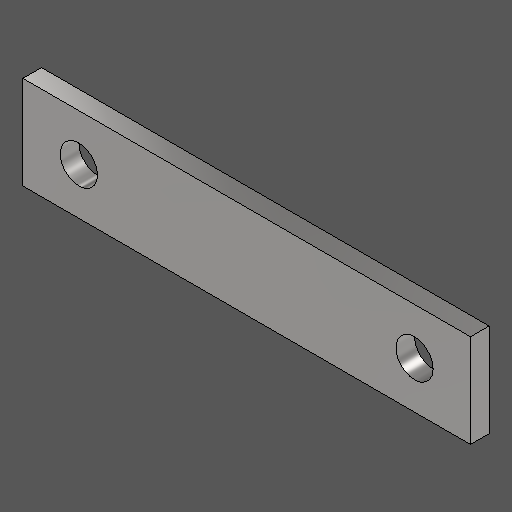
# Autodesk Inventor part: probe-side-large-mesh-support-plate
Saved by Autodesk Inventor 2025 (Build 290162000, 162)
## iProperties
Created: 2024-05-22
Part Number: probe-side-large-mesh-support-plate
Material: Stainless Steel
Document SubType Name: Modeling
Designer: kuzmin
Density: 8 g/cm^3
Appearance: Semi-Polished
Author: kuzmin
Autodesk Inventor part; units mm, degrees
ref_plane "YZ Plane" through (0, 0, 0) normal (1, 0, 0) x (0, 1, 0)
ref_plane "XZ Plane" through (0, 0, 0) normal (0, 1, 0) x (-1, 0, 0)
ref_plane "XY Plane" through (0, 0, 0) normal (0, 0, 1) x (1, 0, 0)
sketch "Sketch1" plane through (0, 0, 0) normal (0, 0, 1) x (1, 0, 0)
  line L0 (-12, 2.5) -> (12, 2.5)
  line L1 (12, 2.5) -> (12, -2.5)
  line L2 (12, -2.5) -> (-12, -2.5)
  line L3 (-12, -2.5) -> (-12, 2.5)
  point P0 (0, 0)
  point P1 (12, 0)
  point P2 (0, 2.5)
  dimension "d0" = 24
  dimension "d1" = 5
  constraints: 8 end point, 2 midpoint, 2 parallel, 1 horizontal, 1 horizontal alignment, 1 perpendicular, 1 vertical alignment
  measures "d0" distance of L0.start L0.end
  measures "d1" distance of L0.end L1.end
extrude "Extrusion1" add sketch "Sketch1" along normal blind 1
sketch "Sketch2" plane through (0, 0, 1) normal (0, 0, 1) x (1, 0, 0)
  line L0 (-9, 0) -> (9, 0) construction
  point P0 (0, 0)
  point P1 (0, 0)
  dimension "d4" = 18
  constraints: 3 coincident, 2 end point, 1 horizontal, 1 midpoint
  measures "d4" distance of L0.start L0.end
hole "Hole1" at (9, 0, 1) at (-9, 0, 1) direction (0, 0, -1) diameter 2 end through all
body "Solid1"
